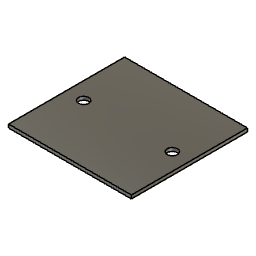
substrate2 (Autodesk Fusion 360 design; units mm, degrees)
Autodesk Fusion 360 part; units mm, degrees
sketch "スケッチ1" plane through (0, 0, 0) normal (0, 0, 1) x (1, 0, 0)
  line L0 (0, 0) -> (36, 0)
  line L1 (36, 0) -> (36, 34)
  line L2 (36, 34) -> (0, 34)
  line L3 (0, 34) -> (0, 0)
  line L4 (0, 34) -> (0, 17)
  line L5 (0, 17) -> (5, 17)
  circle A0 centre (5, 17) radius 1.5
  line L6 (5, 17) -> (31, 17)
  circle A1 centre (31, 17) radius 1.5
  line L7 (31, 17) -> (36, 17)
  dimension "d1" = 36
  dimension "d2" = 34
  dimension "d3" = 3
  dimension "d4" = 26
  dimension "d5" = 3
  constraint horizontal L0
  constraint vertical L1
  constraint horizontal L2
  constraint vertical L3
  constraint coincident L0.start L3.end
  constraint midpoint L3 L4.end
  constraint perpendicular L3 L5
  constraint coincident L5.end A0.centre
  constraint parallel L5 L6
  constraint coincident L6.end A1.centre
  constraint midpoint L1 L7.end
  constraint perpendicular L1 L7
  measures "d1" distance of L0.start L0.end
  measures "d2" distance of L0.start L2.end
  measures "d3" diameter of A0
  measures "d4" distance of L5.end L6.end
  measures "d5" diameter of A1
extrude "押し出し1" add sketch "スケッチ1" along normal blind 1 contours L0 L1 L3 L5 A0 L6 A1 L7 | L1 L2 L3 L4 L5 A0 L6 A1 L7
